Autodesk Inventor part; units mm, degrees
(part 3 of 3)
  line L309 (119.1088, 13.8635) -> (119.1088, 15.39)
  line L310 (119.1088, 15.39) -> (119.1978, 15.39)
  spline S261 degree 2 poles (119.1978, 15.39) (119.798, 14.8268) (121.317, 14.2043) (122.021, 14.2043) knots 0 0 0 1 2 2 2
  spline S262 degree 2 poles (122.021, 14.2043) (123.0288, 14.2043) (124.0588, 15.0417) (124.0588, 15.7308) knots 0 0 0 1 2 2 2
  spline S263 degree 2 poles (124.0588, 15.7308) (124.0588, 16.2792) (123.5178, 16.9609) (122.9324, 17.1313) knots 0 0 0 1 2 2 2
  spline S264 degree 2 poles (122.9324, 17.1313) (122.5101, 17.2499) (121.8061, 17.4129) (121.28, 17.5463) knots 0 0 0 1 2 2 2
  spline S265 degree 2 poles (121.28, 17.5463) (120.8057, 17.6723) (120.0573, 18.0502) (119.7683, 18.354) knots 0 0 0 1 2 2 2
  spline S266 degree 2 poles (119.7683, 18.354) (119.4868, 18.6578) (119.1755, 19.4729) (119.1755, 20.0064) knots 0 0 0 1 2 2 2
  spline S267 degree 2 poles (119.1755, 20.0064) (119.1755, 21.1179) (120.9095, 22.6222) (122.2507, 22.6222) knots 0 0 0 1 2 2 2
  spline S268 degree 2 poles (122.2507, 22.6222) (123.0214, 22.6222) (124.3848, 22.3184) (124.9702, 22.0294) knots 0 0 0 1 2 2 2
  line L311 (124.9702, 22.0294) -> (124.9702, 20.577)
  line L312 (124.9702, 20.577) -> (124.8813, 20.577)
  spline S269 degree 2 poles (124.8813, 20.577) (124.4441, 20.9771) (123.0806, 21.5699) (122.3322, 21.5699) knots 0 0 0 1 2 2 2
  spline S270 degree 2 poles (122.3322, 21.5699) (121.4875, 21.5699) (120.4427, 20.7771) (120.4427, 20.1324) knots 0 0 0 1 2 2 2
  spline S271 degree 2 poles (120.4427, 20.1324) (120.4427, 19.5544) (121.0577, 18.8653) (121.6357, 18.7097) knots 0 0 0 1 2 2 2
  spline S272 degree 2 poles (121.6357, 18.7097) (122.021, 18.6059) (123.1399, 18.3392) (123.5104, 18.228) knots 0 0 0 1 2 2 2
  spline S273 degree 2 poles (123.5104, 18.228) (124.4515, 17.939) (125.3259, 16.7756) (125.3259, 15.9235) knots 0 0 0 1 2 2 2
  spline S274 degree 2 poles (125.3259, 15.9235) (125.3259, 15.3825) (124.8887, 14.3451) (124.496, 13.982) knots 0 0 0 1 2 2 2
  spline S275 degree 2 poles (124.496, 13.982) (124.0588, 13.5819) (122.9473, 13.1521) (122.1099, 13.1521) knots 0 0 0 1 2 2 2
  line L313 (126.5634, 13.3151) -> (126.5634, 22.4591)
  line L314 (126.5634, 22.4591) -> (132.2839, 22.4591)
  line L315 (132.2839, 22.4591) -> (132.2839, 21.3773)
  line L316 (132.2839, 21.3773) -> (127.7786, 21.3773)
  line L317 (127.7786, 21.3773) -> (127.7786, 18.8727)
  line L318 (127.7786, 18.8727) -> (131.9801, 18.8727)
  line L319 (131.9801, 18.8727) -> (131.9801, 17.7908)
  line L320 (131.9801, 17.7908) -> (127.7786, 17.7908)
  line L321 (127.7786, 17.7908) -> (127.7786, 14.397)
  line L322 (127.7786, 14.397) -> (132.2839, 14.397)
  line L323 (132.2839, 14.397) -> (132.2839, 13.3151)
  line L324 (132.2839, 13.3151) -> (126.5634, 13.3151)
  spline S276 degree 2 poles (137.1894, 13.1521) (136.3002, 13.1521) (134.7959, 13.7523) (134.2476, 14.3525) knots 0 0 0 1 2 2 2
  spline S277 degree 2 poles (134.2476, 14.3525) (133.6992, 14.9454) (133.099, 16.7238) (133.099, 17.8797) knots 0 0 0 1 2 2 2
  spline S278 degree 2 poles (133.099, 17.8797) (133.099, 19.0283) (133.6844, 20.7326) (134.2402, 21.3625) knots 0 0 0 1 2 2 2
  spline S279 degree 2 poles (134.2402, 21.3625) (134.7885, 21.9775) (136.2853, 22.6222) (137.2116, 22.6222) knots 0 0 0 1 2 2 2
  spline S280 degree 2 poles (137.2116, 22.6222) (137.671, 22.6222) (138.4787, 22.4888) (138.8196, 22.385) knots 0 0 0 1 2 2 2
  spline S281 degree 2 poles (138.8196, 22.385) (139.116, 22.2887) (139.731, 22.0145) (140.0348, 21.8515) knots 0 0 0 1 2 2 2
  line L325 (140.0348, 21.8515) -> (140.0348, 20.3843)
  line L326 (140.0348, 20.3843) -> (139.9385, 20.3843)
  spline S282 degree 2 poles (139.9385, 20.3843) (139.7755, 20.5325) (139.2716, 20.9475) (138.9085, 21.1476) knots 0 0 0 1 2 2 2
  spline S283 degree 2 poles (138.9085, 21.1476) (138.5602, 21.3402) (137.7377, 21.5848) (137.2042, 21.5848) knots 0 0 0 1 2 2 2
  spline S284 degree 2 poles (137.2042, 21.5848) (136.6188, 21.5848) (135.574, 21.1031) (135.1812, 20.6437) knots 0 0 0 1 2 2 2
  spline S285 degree 2 poles (135.1812, 20.6437) (134.7959, 20.1768) (134.3661, 18.7615) (134.3661, 17.8797) knots 0 0 0 1 2 2 2
  spline S286 degree 2 poles (134.3661, 17.8797) (134.3661, 16.9387) (134.8182, 15.5826) (135.2109, 15.1158) knots 0 0 0 1 2 2 2
  spline S287 degree 2 poles (135.2109, 15.1158) (135.5962, 14.6638) (136.6262, 14.2043) (137.2042, 14.2043) knots 0 0 0 1 2 2 2
  spline S288 degree 2 poles (137.2042, 14.2043) (137.7303, 14.2043) (138.6269, 14.4637) (138.9752, 14.6564) knots 0 0 0 1 2 2 2
  spline S289 degree 2 poles (138.9752, 14.6564) (139.3086, 14.849) (139.8051, 15.2492) (139.9459, 15.39) knots 0 0 0 1 2 2 2
  line L327 (139.9459, 15.39) -> (140.0348, 15.39)
  line L328 (140.0348, 15.39) -> (140.0348, 13.9376)
  spline S290 degree 2 poles (140.0348, 13.9376) (139.731, 13.7968) (139.1975, 13.5374) (138.8196, 13.4189) knots 0 0 0 1 2 2 2
  spline S291 degree 2 poles (138.8196, 13.4189) (138.4194, 13.2855) (137.7377, 13.1521) (137.1894, 13.1521) knots 0 0 0 1 2 2 2
  line L329 (143.3027, 13.3151) -> (143.3027, 21.3773)
  line L330 (143.3027, 21.3773) -> (140.2349, 21.3773)
  line L331 (140.2349, 21.3773) -> (140.2349, 22.4591)
  line L332 (140.2349, 22.4591) -> (147.5857, 22.4591)
  line L333 (147.5857, 22.4591) -> (147.5857, 21.3773)
  line L334 (147.5857, 21.3773) -> (144.5179, 21.3773)
  line L335 (144.5179, 21.3773) -> (144.5179, 13.3151)
  line L336 (144.5179, 13.3151) -> (143.3027, 13.3151)
  line L337 (151.6982, 13.3151) -> (148.1562, 13.3151)
  line L338 (148.1562, 13.3151) -> (148.1562, 14.2488)
  line L339 (148.1562, 14.2488) -> (149.3196, 14.2488)
  line L340 (149.3196, 14.2488) -> (149.3196, 21.5255)
  line L341 (149.3196, 21.5255) -> (148.1562, 21.5255)
  line L342 (148.1562, 21.5255) -> (148.1562, 22.4591)
  line L343 (148.1562, 22.4591) -> (151.6982, 22.4591)
  line L344 (151.6982, 22.4591) -> (151.6982, 21.5255)
  line L345 (151.6982, 21.5255) -> (150.5349, 21.5255)
  line L346 (150.5349, 21.5255) -> (150.5349, 14.2488)
  line L347 (150.5349, 14.2488) -> (151.6982, 14.2488)
  line L348 (151.6982, 14.2488) -> (151.6982, 13.3151)
  spline S292 degree 2 poles (159.6715, 21.4143) (160.1902, 20.8067) (160.7681, 19.0283) (160.7681, 17.8871) knots 0 0 0 1 2 2 2
  spline S293 degree 2 poles (160.7681, 17.8871) (160.7681, 16.7756) (160.205, 14.975) (159.6715, 14.3674) knots 0 0 0 1 2 2 2
  spline S294 degree 2 poles (159.6715, 14.3674) (159.1083, 13.7301) (157.6189, 13.1225) (156.7223, 13.1225) knots 0 0 0 1 2 2 2
  spline S295 degree 2 poles (156.7223, 13.1225) (155.796, 13.1225) (154.314, 13.7523) (153.7731, 14.3674) knots 0 0 0 1 2 2 2
  spline S296 degree 2 poles (153.7731, 14.3674) (153.2469, 14.975) (152.6838, 16.7608) (152.6838, 17.8871) knots 0 0 0 1 2 2 2
  spline S297 degree 2 poles (152.6838, 17.8871) (152.6838, 19.0357) (153.2544, 20.7845) (153.7805, 21.4143) knots 0 0 0 1 2 2 2
  spline S298 degree 2 poles (153.7805, 21.4143) (154.314, 22.0219) (155.8034, 22.6518) (156.7223, 22.6518) knots 0 0 0 1 2 2 2
  spline S299 degree 2 poles (156.7223, 22.6518) (157.6559, 22.6518) (159.1527, 21.9997) (159.6715, 21.4143) knots 0 0 0 1 2 2 2
  spline S300 degree 2 poles (159.501, 17.8871) (159.501, 18.7912) (159.1083, 20.1917) (158.7526, 20.6511) knots 0 0 0 1 2 2 2
  spline S301 degree 2 poles (158.7526, 20.6511) (158.3895, 21.1253) (157.3669, 21.5996) (156.7297, 21.5996) knots 0 0 0 1 2 2 2
  spline S302 degree 2 poles (156.7297, 21.5996) (156.0702, 21.5996) (155.0772, 21.1402) (154.6993, 20.6511) knots 0 0 0 1 2 2 2
  spline S303 degree 2 poles (154.6993, 20.6511) (154.3362, 20.1843) (153.9509, 18.7763) (153.9509, 17.8871) knots 0 0 0 1 2 2 2
  spline S304 degree 2 poles (153.9509, 17.8871) (153.9509, 16.0865) (155.4625, 14.1747) (156.7297, 14.1747) knots 0 0 0 1 2 2 2
  spline S305 degree 2 poles (156.7297, 14.1747) (157.9968, 14.1747) (159.501, 16.0865) (159.501, 17.8871) knots 0 0 0 1 2 2 2
  line L349 (168.645, 13.3151) -> (167.2816, 13.3151)
  line L350 (167.2816, 13.3151) -> (163.2357, 21.1994)
  line L351 (163.2357, 21.1994) -> (163.2357, 13.3151)
  line L352 (163.2357, 13.3151) -> (162.1019, 13.3151)
  line L353 (162.1019, 13.3151) -> (162.1019, 22.4591)
  line L354 (162.1019, 22.4591) -> (163.8285, 22.4591)
  line L355 (163.8285, 22.4591) -> (167.5113, 15.2195)
  line L356 (167.5113, 15.2195) -> (167.5113, 22.4591)
  line L357 (167.5113, 22.4591) -> (168.645, 22.4591)
  line L358 (168.645, 22.4591) -> (168.645, 13.3151)
  spline S306 degree 2 poles (180.6271, 16.1236) (180.6271, 15.4418) (180.1084, 14.397) (179.6786, 14.0561) knots 0 0 0 1 2 2 2
  spline S307 degree 2 poles (179.6786, 14.0561) (179.1599, 13.656) (177.9817, 13.3151) (177.048, 13.3151) knots 0 0 0 1 2 2 2
  line L359 (177.048, 13.3151) -> (174.4249, 13.3151)
  line L360 (174.4249, 13.3151) -> (174.4249, 22.4591)
  line L361 (174.4249, 22.4591) -> (176.8479, 22.4591)
  spline S308 degree 2 poles (176.8479, 22.4591) (177.8261, 22.4591) (178.8042, 22.3332) (179.2488, 22.0886) knots 0 0 0 1 2 2 2
  spline S309 degree 2 poles (179.2488, 22.0886) (179.7453, 21.8293) (180.1973, 20.9771) (180.1973, 20.3991) knots 0 0 0 1 2 2 2
  spline S310 degree 2 poles (180.1973, 20.3991) (180.1973, 19.7545) (179.5156, 18.7319) (178.9153, 18.4429) knots 0 0 0 1 2 2 2
  line L362 (178.9153, 18.4429) -> (178.9153, 18.3984)
  spline S311 degree 2 poles (178.9153, 18.3984) (179.7305, 18.1761) (180.6271, 16.9979) (180.6271, 16.1236) knots 0 0 0 1 2 2 2
  spline S312 degree 2 poles (179.36, 16.0717) (179.36, 16.5904) (179.0636, 17.2573) (178.6189, 17.4944) knots 0 0 0 1 2 2 2
  spline S313 degree 2 poles (178.6189, 17.4944) (178.33, 17.6426) (177.6482, 17.7315) (177.0184, 17.7315) knots 0 0 0 1 2 2 2
  line L363 (177.0184, 17.7315) -> (175.6401, 17.7315)
  line L364 (175.6401, 17.7315) -> (175.6401, 14.3525)
  line L365 (175.6401, 14.3525) -> (176.6256, 14.3525)
  spline S314 degree 2 poles (176.6256, 14.3525) (177.4259, 14.3525) (178.3448, 14.5008) (178.7005, 14.7379) knots 0 0 0 1 2 2 2
  spline S315 degree 2 poles (178.7005, 14.7379) (179.0413, 14.9824) (179.36, 15.59) (179.36, 16.0717) knots 0 0 0 1 2 2 2
  spline S316 degree 2 poles (178.9302, 20.2287) (178.9302, 20.5548) (178.7079, 21.0438) (178.4633, 21.1846) knots 0 0 0 1 2 2 2
  spline S317 degree 2 poles (178.4633, 21.1846) (178.1669, 21.3476) (177.4482, 21.4217) (176.8035, 21.4217) knots 0 0 0 1 2 2 2
  line L366 (176.8035, 21.4217) -> (175.6401, 21.4217)
  line L367 (175.6401, 21.4217) -> (175.6401, 18.7467)
  line L368 (175.6401, 18.7467) -> (177.0184, 18.7467)
  spline S318 degree 2 poles (177.0184, 18.7467) (177.589, 18.7467) (178.1299, 18.8653) (178.4189, 19.0505) knots 0 0 0 1 2 2 2
  spline S319 degree 2 poles (178.4189, 19.0505) (178.7005, 19.2284) (178.9302, 19.7989) (178.9302, 20.2287) knots 0 0 0 1 2 2 2
  spline S320 degree 2 poles (187.2665, 17.8871) (187.2665, 15.427) (185.8363, 13.1225) (184.3469, 13.1225) knots 0 0 0 1 2 2 2
  spline S321 degree 2 poles (184.3469, 13.1225) (182.8353, 13.1225) (181.4199, 15.4715) (181.4199, 17.8797) knots 0 0 0 1 2 2 2
  spline S322 degree 2 poles (181.4199, 17.8797) (181.4199, 20.3547) (182.8501, 22.6444) (184.3469, 22.6444) knots 0 0 0 1 2 2 2
  spline S323 degree 2 poles (184.3469, 22.6444) (185.8512, 22.6444) (187.2665, 20.2732) (187.2665, 17.8871) knots 0 0 0 1 2 2 2
  spline S324 degree 2 poles (185.6955, 15.101) (185.8734, 15.553) (186.0216, 16.9461) (186.0216, 17.8871) knots 0 0 0 1 2 2 2
  spline S325 degree 2 poles (186.0216, 17.8871) (186.0216, 18.8282) (185.8734, 20.2139) (185.6881, 20.6807) knots 0 0 0 1 2 2 2
  spline S326 degree 2 poles (185.6881, 20.6807) (185.5029, 21.1476) (184.8582, 21.6292) (184.3469, 21.6292) knots 0 0 0 1 2 2 2
  spline S327 degree 2 poles (184.3469, 21.6292) (183.8356, 21.6292) (183.1761, 21.1476) (182.9835, 20.6659) knots 0 0 0 1 2 2 2
  spline S328 degree 2 poles (182.9835, 20.6659) (182.7982, 20.1991) (182.6648, 18.7763) (182.6648, 17.8797) knots 0 0 0 1 2 2 2
  spline S329 degree 2 poles (182.6648, 17.8797) (182.6648, 16.9164) (182.7834, 15.6271) (182.9761, 15.1232) knots 0 0 0 1 2 2 2
  spline S330 degree 2 poles (182.9761, 15.1232) (183.1539, 14.649) (183.8134, 14.1377) (184.3469, 14.1377) knots 0 0 0 1 2 2 2
  spline S331 degree 2 poles (184.3469, 14.1377) (184.8508, 14.1377) (185.5103, 14.6193) (185.6955, 15.101) knots 0 0 0 1 2 2 2
  spline S332 degree 2 poles (190.9048, 21.5922) (190.5714, 21.5922) (189.9119, 21.4291) (189.5932, 21.3032) knots 0 0 0 1 2 2 2
  spline S333 degree 2 poles (189.5932, 21.3032) (189.2968, 21.1772) (188.8596, 20.9104) (188.6892, 20.7919) knots 0 0 0 1 2 2 2
  line L369 (188.6892, 20.7919) -> (188.6151, 20.7919)
  line L370 (188.6151, 20.7919) -> (188.6151, 22.0886)
  spline S334 degree 2 poles (188.6151, 22.0886) (189.0152, 22.3035) (190.3861, 22.6518) (191.0011, 22.6518) knots 0 0 0 1 2 2 2
  spline S335 degree 2 poles (191.0011, 22.6518) (191.6236, 22.6518) (192.5498, 22.3999) (192.9278, 22.1331) knots 0 0 0 1 2 2 2
  spline S336 degree 2 poles (192.9278, 22.1331) (193.3279, 21.8441) (193.7429, 21.0068) (193.7429, 20.4436) knots 0 0 0 1 2 2 2
  spline S337 degree 2 poles (193.7429, 20.4436) (193.7429, 19.6878) (192.7499, 18.5466) (192.0534, 18.3984) knots 0 0 0 1 2 2 2
  line L371 (192.0534, 18.3984) -> (192.0534, 18.3095)
  spline S338 degree 2 poles (192.0534, 18.3095) (192.3424, 18.2502) (193.0019, 17.9835) (193.2834, 17.7167) knots 0 0 0 1 2 2 2
  spline S339 degree 2 poles (193.2834, 17.7167) (193.565, 17.4574) (193.9207, 16.6274) (193.9207, 16.0272) knots 0 0 0 1 2 2 2
  spline S340 degree 2 poles (193.9207, 16.0272) (193.9207, 15.4122) (193.4983, 14.3674) (193.113, 13.9672) knots 0 0 0 1 2 2 2
  spline S341 degree 2 poles (193.113, 13.9672) (192.7129, 13.5523) (191.5791, 13.1225) (190.8603, 13.1225) knots 0 0 0 1 2 2 2
  spline S342 degree 2 poles (190.8603, 13.1225) (190.1712, 13.1225) (188.8226, 13.4559) (188.3632, 13.6856) knots 0 0 0 1 2 2 2
  line L372 (188.3632, 13.6856) -> (188.3632, 14.9824)
  line L373 (188.3632, 14.9824) -> (188.4521, 14.9824)
  spline S343 degree 2 poles (188.4521, 14.9824) (188.8374, 14.7008) (190.1416, 14.1821) (190.7862, 14.1821) knots 0 0 0 1 2 2 2
  spline S344 degree 2 poles (190.7862, 14.1821) (191.1642, 14.1821) (191.92, 14.4192) (192.1719, 14.6934) knots 0 0 0 1 2 2 2
  spline S345 degree 2 poles (192.1719, 14.6934) (192.4165, 14.9676) (192.6758, 15.6197) (192.6758, 16.1161) knots 0 0 0 1 2 2 2
  spline S346 degree 2 poles (192.6758, 16.1161) (192.6758, 16.6126) (192.3868, 17.2573) (192.1275, 17.4425) knots 0 0 0 1 2 2 2
  spline S347 degree 2 poles (192.1275, 17.4425) (191.8681, 17.6278) (191.1642, 17.7686) (190.7492, 17.7686) knots 0 0 0 1 2 2 2
  line L374 (190.7492, 17.7686) -> (190.2305, 17.7686)
  line L375 (190.2305, 17.7686) -> (190.2305, 18.7838)
  line L376 (190.2305, 18.7838) -> (190.638, 18.7838)
  spline S348 degree 2 poles (190.638, 18.7838) (191.4606, 18.7838) (192.498, 19.5692) (192.498, 20.3176) knots 0 0 0 1 2 2 2
  spline S349 degree 2 poles (192.498, 20.3176) (192.498, 20.6659) (192.2312, 21.1624) (192.0163, 21.3106) knots 0 0 0 1 2 2 2
  spline S350 degree 2 poles (192.0163, 21.3106) (191.7866, 21.4662) (191.2234, 21.5922) (190.9048, 21.5922) knots 0 0 0 1 2 2 2
  dimension "d25" = 203.2
  dimension "d26" = 50.8
  dimension "d27" = 45.72
  dimension "d28" = 2.54
  dimension "d29" = 8.4667
  dimension "d30" = 101.6
  dimension "d31" = 76.2
  dimension "d32" = 12.7
  dimension "d33" = 25.4
  dimension "d34" = 8.4667
  constraints: 4 other
  measures "d25" distance of L1.start L1.end
  measures "d26" distance of L1.end L0.start
  measures "d27" distance of L6.end L4.start
  measures "d28" distance between parallel lines of L1 L4
  measures "d29" distance between parallel lines of L2 L7
  measures "d30" distance of L4.start L4.end
  measures "d31" distance of L8.start L8.end
  measures "d32" distance between parallel lines of L1 L8
  measures "d33" distance of L8.end L9.end
  measures "d34" distance between parallel lines of L5 L11
extrude "Extrusion5" cut sketch "Sketch5" against normal blind 5.08 contours S0 S1 L12 L13 S2 S3 S4 L14 L15 L16 L17 L18 | S5 S6 L19 L20 L21 S7 S8 S9 S10 L22 L23 L24 S11 S12 | S13 L25 L26 S14 S15 S16 S17 S18 S19 S20 S21 L27 L28 S22 S23 S24 S25 S26 S27 S28 | L29 L30 L31 L32 L33 L34 L35 L36 | L37 L38 L39 L40 L41 L42 L43 L44 L45 L46 L47 L48 | L49 L50 L51 L52 L53 L54 L55 L56 L57 L58 | L59 L60 L61 L62 L63 L64 L65 L66 | L70 L71 L72 L73 L74 L75 | L76 L77 L78 L79 L80 L81 | L82 L83 L84 L85 L86 L87 L88 L89 L90 L91 L92 L93 | L94 L95 L96 L97 L98 L99 L100 L101 L102 L103 | L104 L105 L106 L107 L108 L109 L110 L111 | L115 L116 L117 L118 L119 L120 S29 L121 L122 L123 L124 | L125 L126 L127 L128 L129 L130 L131 L132 L133 L134 L135 | S30 S31 S32 L139 L140 S33 S34 S35 S36 S37 S38 S39 L141 L142 L143 L144 L145 S40 S41 S42 | S43 S44 S45 S46 S47 S48 S49 L146 L147 S50 S51 S52 S53 S54 | S62 S63 S64 S65 S66 S67 S68 L148 L149 S69 S70 S71 S72 S73 | S81 S82 S83 S84 | L150 L151 L152 L153 L154 L155 L156 | L157 L158 L159 L160 L161 L162 S93 L163 L164 L165 L166 | S94 S95 L167 L168 S96 S97 S98 L169 L170 L171 L172 L173 | L174 L175 L176 L177 | S99 S100 L178 L179 L180 L181 L182 S101 S102 | S107 S108 S109 S110 S111 S112 L184 S113 S114 S115 L185 L186 S116 S117 S118 L187 L188 L189 | L191 L192 L193 L194 | L195 L196 L197 L198 | S123 S124 S125 S126 L199 L200 S127 S128 S129 L201 L202 S130 S131 | L204 L205 S136 S137 S138 L206 L207 L208 L209 L210 S139 S140 L211 | S141 L212 L213 S142 S143 S144 S145 L214 L215 L216 L217 S146 S147 S148 S149 S150 L218 S151 S152 S153 S154 | L220 L221 S159 S160 S161 L222 L223 L224 S162 S163 S164 L225 L226 L227 | S165 S166 S167 S168 S169 L228 L229 S170 S171 S172 S173 S174 L230 L231 S175 S176 | S177 L232 L233 S178 S179 S180 S181 S182 S183 S184 S185 S186 L234 L235 S187 S188 S189 S190 S191 S192 S193 | L236 L237 S194 S195 S196 S197 S198 S199 S200 L238 L239 L240 | L242 L243 L244 L245 | S205 S206 S207 S208 L246 L247 S209 S210 S211 L248 L249 S212 S213 | L251 L252 S218 S219 S220 S221 S222 S223 S224 L253 L254 L255 | L257 L258 S229 S230 S231 L259 L260 L261 S232 S233 S234 L262 L263 L264 | L265 L266 L267 L268 L269 L270 L271 L272 L273 L274 L275 L276 L277 | S235 S236 L278 L279 L280 S237 S238 S239 S240 L281 L282 L283 S241 S242 | S243 L284 L285 S244 S245 S246 S247 S248 S249 S250 S251 L286 L287 S252 S253 S254 S255 S256 S257 S258 | L288 L289 L290 L291 L292 L293 S259 L294 L295 L296 L297 | L298 L299 L300 L301 L302 L303 L304 L305 | S260 L309 L310 S261 S262 S263 S264 S265 S266 S267 S268 L311 L312 S269 S270 S271 S272 S273 S274 S275 | L313 L314 L315 L316 L317 L318 L319 L320 L321 L322 L323 L324 | S276 S277 S278 S279 S280 S281 L325 L326 S282 S283 S284 S285 S286 S287 S288 S289 L327 L328 S290 S291 | L329 L330 L331 L332 L333 L334 L335 L336 | L337 L338 L339 L340 L341 L342 L343 L344 L345 L346 L347 L348 | S292 S293 S294 S295 S296 S297 S298 S299 | L349 L350 L351 L352 L353 L354 L355 L356 L357 L358 | S306 S307 L359 L360 L361 S308 S309 S310 L362 S311 | S320 S321 S322 S323 | S332 S333 L369 L370 S334 S335 S336 S337 L371 S338 S339 S340 S341 S342 L372 L373 S343 S344 S345 S346 S347 L374 L375 L376 S348 S349 S350
equation "\"d6\" = 0.5 * d3 - 0.5 * d5"
equation "\"d7\" = 0.5 * d2 - 0.5 * d4"
equation "\"d14\" = 0.5 * d10 - 0.5 * d12"
equation "\"d15\" = 0.5 * d11 - 0.5 * d13"
equation "\"d22\" = 0.5 * d21 - 0.5 * d19"
equation "\"d28\" = 0.5 * d26 - 0.5 * d27"
equation "\"d29\" = -0.333333 * d31 + 0.333333 * d25 - 0.333333 * d30"
equation "\"d32\" = 0.5 * d26 - 0.5 * d33"
equation "\"d34\" = d29"
body "Solid1"
